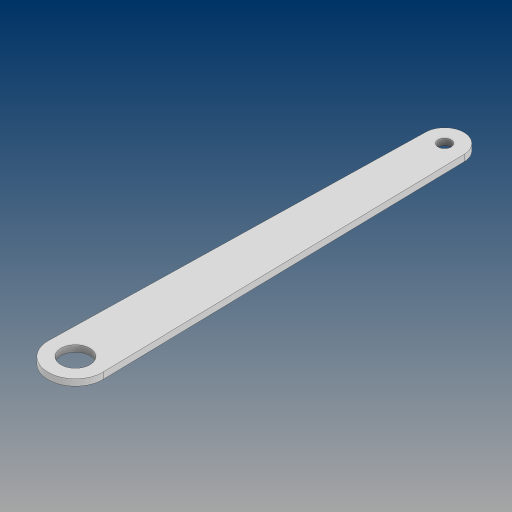
# Autodesk Inventor part: DragBarLinkage3 Bar3
Saved by Autodesk Inventor 2024.3 (Build 283343000, 343)
## iProperties
Created: 2024-07-08
Part Number: DragBarLinkage3 Bar3
Material: Generic
Document SubType Name: Modeling
Designer: Kenji
Density: 1 g/cm^3
Appearance: Default
Author: Kenji
Autodesk Inventor part; units mm, degrees
ref_plane "YZ Plane" through (0, 0, 0) normal (1, 0, 0) x (0, 1, 0)
ref_plane "XZ Plane" through (0, 0, 0) normal (0, 1, 0) x (-1, 0, 0)
ref_plane "XY Plane" through (0, 0, 0) normal (0, 0, 1) x (1, 0, 0)
sketch "Sketch1" plane through (0, 0, 0) normal (0, 1, 0) x (-1, 0, 0)
  line L0 (0, 0) -> (0, -365.76) construction
  circle A0 centre (0, -365.76) radius 6.35
  circle A1 centre (0, 0) radius 14.2875
  circle A2 centre (0, 0) radius 26.9875 construction
  circle A3 centre (0, -365.76) radius 19.05 construction
  line L1 (26.9811, -0.5857) -> (19.0455, -366.1734)
  line L2 (-19.0455, -366.1734) -> (-26.9811, -0.5857)
  arc A4 (26.9811, -0.5857) -> (-26.9811, -0.5857) centre (0, 0) ccw
  arc A5 (-12.3767, -351.2783) -> (19.0455, -366.1734) centre (0, -365.76) ccw
  dimension "d0" = 365.76
  dimension "d1" = 12.7
  dimension "d2" = 28.575
  dimension "d3" = 12.7
  dimension "d4" = 12.7
  constraints: 9 point on circle, 6 centre point, 6 end point, 6 tangent, 2 coincident, 1 concentric, 1 vertical
  measures "d0" distance of L0.start L0.end
  measures "d1" diameter of A0
  measures "d2" diameter of A1
  measures "d3" radial gap between concentric circles of A1 A2
  measures "d4" radial gap between concentric circles of A0 A3
extrude "Extrusion1" add sketch "Sketch1" along normal blind 6.35
body "Solid1"
